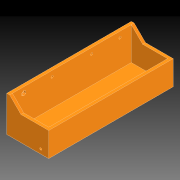
# Autodesk Inventor part: KB33-046-008-001 - Корпус
Saved by Autodesk Inventor 2020 (Build 240168000, 168)
## iProperties
Created: 2021-08-09
Part Number: KB33-046-008-001 - Корпус
Material: Типовые
Document SubType Name: Modeling
Designer: Петров Иван
Mass: 212.866 g
Surface Area: 886.123 cm^2
Volume: 212.866 cm^3
Density: 1 g/cm^3
Appearance: Оранжевый
Author: Петров Иван
Autodesk Inventor part; units mm, degrees
ref_plane "YZ Plane" through (0, 0, 0) normal (1, 0, 0) x (0, 1, 0)
ref_plane "XZ Plane" through (0, 0, 0) normal (0, 1, 0) x (-1, 0, 0)
ref_plane "XY Plane" through (0, 0, 0) normal (0, 0, 1) x (1, 0, 0)
sketch "Эскиз1" plane through (0, 0, 0) normal (0, 1, 0) x (-1, 0, 0)
  line L0 (-37, 110) -> (37, 110)
  line L1 (37, 110) -> (37, -110)
  line L2 (37, -110) -> (-37, -110)
  line L3 (-37, -110) -> (-37, 110)
  line L4 (-37, 110) -> (37, -110) construction
  line L5 (37, 110) -> (-37, -110) construction
  point P0 (0, 0)
  dimension "d0" = 74
  dimension "d1" = 220
  constraints: 12 end point, 2 midpoint, 2 parallel, 1 horizontal, 1 perpendicular
  measures "d0" distance of L1.end L2.end
  measures "d1" distance of L0.end L1.end
extrude "Выдавливание1" add sketch "Эскиз1" along normal blind 43
sketch "Эскиз3" plane through (0, 43, 0) normal (0, 1, 0) x (1, 0, 0)
  line L0 (-32, -105) -> (32, -105)
  line L1 (32, -105) -> (32, 105)
  line L2 (32, 105) -> (-32, 105)
  line L3 (-32, 105) -> (-32, -105)
  line L4 (-32, -105) -> (32, 105) construction
  line L5 (32, -105) -> (-32, 105) construction
  line L6 (37, 110) -> (-37, 110) projected
  line L7 (-37, 110) -> (-37, -110) projected
  point P0 (0, 0)
  dimension "d4" = 5
  dimension "d5" = 5
  constraints: 12 end point, 2 midpoint, 2 parallel, 1 horizontal, 1 perpendicular
  measures "d4" distance between parallel lines of L6 L2
  measures "d5" distance between parallel lines of L7 L3
extrude "Выдавливание2" cut sketch "Эскиз3" against normal blind 38
sketch "Эскиз4" plane through (0, 5, 0) normal (0, 1, 0) x (1, 0, 0)
  line L0 (32, 105) -> (32, -105) projected
  line L1 (32, 105) -> (0, 105)
  line L2 (0, 105) -> (0, 67.1211)
  line L3 (0, 67.1211) -> (32, 67.1211)
  line L4 (32, 67.1211) -> (32, 105)
  point P0 (0, 0)
  constraints: 8 end point, 2 parallel, 1 horizontal, 1 perpendicular
sketch "Эскиз5" plane through (0, 43, 0) normal (0, 1, 0) x (1, 0, 0)
  line L0 (-37, 110) -> (-37, -110) projected
  line L1 (-37, -110) -> (37, -110) projected
  line L2 (-37, 110) -> (-32, 110)
  line L3 (-32, 110) -> (-32, -110)
  line L4 (-32, -110) -> (-37, -110)
  line L5 (-37, -110) -> (-37, 110)
  line L6 (-32, -105) -> (-32, 105) projected
  point P0 (0, 0)
  point P1 (-32, 0)
  constraints: 8 end point, 2 midpoint, 2 parallel, 1 horizontal, 1 perpendicular, 1 point on line
extrude "Выдавливание3" add sketch "Эскиз5" along normal blind 20
chamfer "Фаска1" distance 20 angle 45 2 edges at (-32, 43, -107.5) (-32, 43, 107.5)
sketch "Эскиз6" plane through (-37, 0, -110) normal (-1, 0, 0) x (0, 0, 1)
  circle A0 centre (25, 53) radius 2
  circle A1 centre (75, 53) radius 2
  line L0 (0, 63) -> (220, 63) projected
  point P0 (110, 0)
  dimension "d13" = 4
  dimension "d14" = 4
  dimension "d15" = 10
  dimension "d16" = 50
  dimension "d19" = 35
  constraints: 2 centre point, 1 horizontal alignment
  measures "d13" diameter of A0
  measures "d14" diameter of A1
  measures "d15" distance from line of L0 A1.centre
  measures "d16" distance of A0.centre A1.centre
  measures "d19" horizontal distance of point (110, 0) A1.centre
extrude "Выдавливание4" cut sketch "Эскиз6" against normal blind 10
mirror "Зеркальное отражение1" about plane through (0, 0, 0) normal (0, 0, 1) of "Выдавливание4"
sketch "Эскиз7" plane through (-37, 0, 110) normal (0, 0, 1) x (1, 0, 0)
  circle A0 centre (59.9136, 7.71) radius 1.85 projected
  point P0 (37, 0)
extrude "Выдавливание5" cut sketch "Эскиз7" against normal through all
sketch "Эскиз8" plane through (-32, 5, 105) normal (1, 0, 0) x (0, 0, -1)
  circle A0 centre (20, 48) radius 2 projected
  line L0 (20, 52.0415) -> (23.5, 50.0207)
  line L1 (23.5, 50.0207) -> (23.5, 45.9793)
  line L2 (23.5, 45.9793) -> (20, 43.9585)
  line L3 (20, 43.9585) -> (16.5, 45.9793)
  line L4 (16.5, 45.9793) -> (16.5, 50.0207)
  line L5 (16.5, 50.0207) -> (20, 52.0415)
  point P0 (105, -5)
  dimension "d22" = 7
  constraints: 12 end point, 1 coincident, 13 other
  measures "d22" distance between parallel lines of L4 L1
extrude "Выдавливание6" cut sketch "Эскиз8" against normal blind 3.2 contours A0 | L0 L1 L2 L3 L4 L5
